Dog Game (Autodesk Fusion 360 design; units mm, degrees)
description: Spur Gear; Module: 1.5; Num Teeth: 32; Pressure Angle: 20.0; Backlash: 0.15 mm
description: Spur Gear; Module: 1.5; Num Teeth: 16; Pressure Angle: 20.0; Backlash: 0.15 mm
Autodesk Fusion 360 part; units mm, degrees
sketch "Sketch1" plane through (0, 0, 0) normal (0, 0, 1) x (1, 0, 0) in component "Pipe"
  arc A0 (120, 0) -> (-43.6285, 111.788) centre (0, 0) ccw
  dimension "d9" = 120
  constraint coincident A0.centre origin
  measures "d9" radius of A0
pipe "Pipe1" add diameter 91 wall 3 path "Sketch1" along A0 makes body 1 in component "Pipe"
sketch "Sketch1 (2)" plane through (0, 0, 0) normal (0, 1, 0) x (1, 0, 0) in component "Wheel"
  circle A0 centre (0, -56.6188) radius 34
  line L0 (-12.5, -25) -> (12.5, -25)
  line L1 (-12.5, -15) -> (12.5, -15)
  line L2 (12.5, -15) -> (12.5, -5)
  line L3 (12.5, -5) -> (-12.5, -5)
  line L4 (-12.5, -5) -> (-12.5, -15)
  line L5 (-12.5, -15) -> (12.5, -5) construction
  line L6 (12.5, -15) -> (-12.5, -5) construction
  line L7 (-9.5, -15) -> (-8.0858, -13.5858)
  line L8 (-9.5, -15) -> (-6.1258, -15) construction
  line L9 (9.5, -15) -> (8.0858, -13.5858)
  line L10 (9.5, -15) -> (10.773, -15) construction
  line L11 (-8.0858, -13.5858) -> (8.0858, -13.5858)
  line L12 (-1.4142, -13.5858) -> (0, -12.1716)
  line L13 (-1.4142, -13.5858) -> (0.8453, -13.5858) construction
  line L14 (0, 0) -> (0, -140)
  line L15 (1.4142, -13.5858) -> (0, -12.1716)
  line L16 (1.4142, -13.5858) -> (3.4142, -13.5858) construction
  arc A1 (12.5, -25) -> (12.5, -15) centre (8.3467, -20) ccw
  line L17 (12.5, -5) -> (-12.5, -5)
  line L18 (-12.5, -5) -> (-12.5, 0)
  line L19 (-12.5, 0) -> (12.5, 0)
  line L20 (12.5, 0) -> (12.5, -5)
  arc A2 (-12.5, -15) -> (-12.5, -25) centre (-8.3467, -20) ccw
  point P0 (0, -10)
  dimension "d40" = 68
  dimension "d42" = 25
  dimension "d43" = 25
  dimension "d45" = 45
  dimension "d46" = 2
  dimension "d47" = 3
  dimension "d48" = 135
  dimension "d49" = 2
  dimension "d50" = 3
  dimension "d51" = 2
  dimension "d52" = 45
  dimension "d53" = 140
  dimension "d54" = 135
  dimension "d55" = 2
  dimension "d60" = 10
  dimension "d61" = 5
  dimension "d62" = 6.5
  dimension "d64" = 10
  dimension "d65" = 6.5
  constraint horizontal L0
  constraint coincident A0 L0.start
  constraint coincident A0 L0.end
  constraint horizontal L1
  constraint perpendicular L1 L2
  constraint parallel L1 L3
  constraint parallel L2 L4
  constraint coincident L5 P0
  constraint coincident L6 P0
  constraint vertical L14.start P0
  constraint horizontal L8
  constraint coincident L1 L7.start
  constraint horizontal L10
  constraint coincident L1 L9.start
  constraint horizontal L13
  constraint coincident L11 L12.start
  constraint vertical L14
  constraint coincident L14.start origin
  constraint coincident L12.end L14
  constraint horizontal L16
  constraint coincident L11 L15.start
  constraint coincident L14 L12.end
  constraint coincident A0.centre L14
  constraint horizontal L17
  constraint vertical L18
  constraint horizontal L19
  constraint vertical L20
  constraint coincident L14.start L19
  measures "d40" diameter of A0
  measures "d42" distance of L0.start L0.end
  measures "d43" distance of L2.end L3.end
  measures "d45" angle of L7 L8
  measures "d46" distance of L7.start L7.end
  measures "d47" distance of L1.start L7.start
  measures "d48" angle of L9 L10
  measures "d49" distance of L9.start L9.end
  measures "d50" distance of L1.end L9.start
  measures "d51" distance of L12.start L12.end
  measures "d52" angle of L12 L13
  measures "d53" distance of L14.start L14.end
  measures "d54" angle of L15 L16
  measures "d55" distance of L15.start L12.end
  measures "d60" distance of L0 L1
  measures "d61" distance of L2.end L19.end
  measures "d62" radius of A1
  measures "d64" distance of L1.start L3.end
  measures "d65" radius of A2
revolve "Revolve1" add sketch "Sketch1 (2)" angle 360 about axis through (1.75, 0, 0) along (1, 0, 0) separate body contours L1 L2 L3 L9 L11 L14 L15 L17 | L3 L14 L17 L19 L20 | L1 L3 L4 L7 L11 L12 L14 L17 | L3 L14 L17 L18 L19 makes body 2 in component "Wheel"
revolve "Revolve2" add sketch "Sketch1 (2)" angle 360 about axis through (1.75, 0, 0) along (1, 0, 0) separate body contours A0 L1 L14 A1 | A0 L1 L14 A2 | L1 L9 L11 L14 | L1 L7 L11 L14 | L11 L14 L15 | L11 L12 L14 makes body 3 in component "Wheel"
fillet "Fillet1" radius 4.5 2 edges at (12.5, -9.0404, -23.3082) (-12.5, -9.0404, -23.3082) on bodies 3 in component "Wheel"
sketch "Sketch2" plane through (12.5, 0, 0) normal (1, 0, 0) x (0, 1, 0) in component "Wheel"
  circle A0 centre (0, 0) radius 15
  circle A1 centre (0, 0) radius 4
  circle A2 centre (0, 0) radius 7.5
  dimension "d68" = 8
  dimension "d69" = 15
  constraint concentric A0 A1
  constraint concentric A0 A2
  measures "d68" diameter of A1
  measures "d69" diameter of A2
extrude "Extrude1" cut sketch "Sketch2" against normal blind 40 contours A1 bodies 2 in component "Wheel"
extrude "Extrude2" add sketch "Sketch2" along normal blind 10 contours A2 bodies 2 in component "Wheel"
sketch "Sketch3" plane through (0, 0, 0) normal (0, 1, 0) x (1, 0, 0) in component "Wheel"
  line L0 (20, -2.5) -> (15, -2.5)
  line L1 (15, -2.5) -> (15, 2.5)
  line L2 (15, 2.5) -> (20, 2.5)
  line L3 (20, 2.5) -> (20, -2.5)
  line L4 (22.5, -7.5) -> (22.5, 7.5)
  circle A0 centre (17.5, 0) radius 1.5
  line L5 (0, 0) -> (31.5, 0)
  dimension "d74" = 5
  dimension "d75" = 5
  dimension "d76" = 2.5
  dimension "d77" = 3
  dimension "d85" = 2.5
  dimension "d86" = 2.5
  constraint horizontal L0
  constraint vertical L1
  constraint horizontal L2
  constraint vertical L3
  constraint coincident L5.start origin
  constraint perpendicular L3 L5
  constraint coincident A0.centre L5
  measures "d74" distance of L0.start L0.end
  measures "d75" distance of L0.start L2.end
  measures "d76" distance of L3 L4
  measures "d77" diameter of A0
  measures "d85" distance of L0 L5
  measures "d86" distance of L1 A0.centre
extrude "Extrude3" cut sketch "Sketch3" along normal blind 2 from surface at 6.7 bodies 2 in component "Wheel"
extrude "Extrude4" cut sketch "Sketch3" along normal blind 2 from surface at -8.7 bodies 2 in component "Wheel"
extrude "Extrude5" cut sketch "Sketch3" along normal mid plane 40 contours A0 L5 | A0 L5 bodies 2 in component "Wheel"
fillet "Fillet2" radius 2.5 1 edges at (12.5, -6.9925, 2.7121) on bodies 2 in component "Wheel"
sketch "Sketch1 (3)" plane through (0, 0, 0) normal (0, 0, 1) x (1, 0, 0) in component "Motor Connection"
  circle A0 centre (0, 0) radius 3.75
  circle A1 centre (0, 0) radius 6
  line L0 (-20.0347, 2.5) -> (19.9653, 2.5)
  line L1 (-1, 0) -> (1, 0)
  line L2 (1, 0) -> (1, -13.1685)
  line L3 (1, -13.1685) -> (-1, -13.1685)
  line L4 (-1, -13.1685) -> (-1, 0)
  circle A2 centre (0, 0) radius 4
  dimension "d1_1" = 7.5
  dimension "d2_1" = 12
  dimension "d3_1" = 40
  dimension "d4_1" = 2.5
  dimension "d5_1" = 2
  dimension "d95" = 8
  constraint coincident A0.centre A1.centre
  constraint horizontal L0
  constraint horizontal L1
  constraint vertical L2
  constraint horizontal L3
  constraint vertical L4
  constraint midpoint A0.centre L1
  measures "d1_1" diameter of A0
  measures "d2_1" diameter of A1
  measures "d3_1" distance of L0.start L0.end
  measures "d4_1" distance of A0.centre L0
  measures "d5_1" distance of L2.end L3.end
  measures "d95" diameter of A2
extrude "Extrude1'" add sketch "Sketch1 (3)" along normal blind 12.5 separate body contours A0 L0 L2 A2 | A0 L0 | A0 L0 A2 | A0 L0 L4 A2 | A1 L0 A2 | A1 L0 L2 A2 | A1 L0 L4 A2 makes body 4 in component "Motor Connection"
extrude "Extrude9" add sketch "Sketch1 (3)" along normal blind 12 from surface at 12 contours A1 L0 A2 | A1 L0 L2 A2 | A1 L0 L4 A2 bodies 4 in component "Motor Connection"
sketch "Sketch4" plane through (0, 0, 0) normal (1, 0, 0) x (0, 1, 0) in component "Motor Connection"
  line L0 (2.5, 20.5) -> (-2.5, 20.5)
  line L1 (-2.5, 20.5) -> (-2.5, 15.5)
  line L2 (-2.5, 15.5) -> (2.5, 15.5)
  line L3 (2.5, 15.5) -> (2.5, 20.5)
  line L4 (2.5, 20.5) -> (-2.5, 15.5) construction
  line L5 (-2.5, 20.5) -> (2.5, 15.5) construction
  line L6 (6, 24) -> (-5.9161, 24)
  circle A0 centre (0, 18) radius 1.5
  point P0 (0, 18)
  dimension "d99" = 5
  dimension "d100" = 5
  dimension "d101" = 3.5
  dimension "d102" = 3
  constraint horizontal L0
  constraint perpendicular L0 L1
  constraint parallel L0 L2
  constraint parallel L1 L3
  constraint coincident L4 P0
  constraint coincident L5 P0
  constraint coincident P0 A0.centre
  measures "d99" distance of L1.end L2.end
  measures "d100" distance of L0.end L1.end
  measures "d101" distance of L0 L6
  measures "d102" diameter of A0
extrude "Extrude10" cut sketch "Sketch4" along normal blind 2 from surface at 5.3 contours L0 L1 L2 L3 | A0 bodies 4 in component "Motor Connection"
extrude "Extrude11" cut sketch "Sketch4" along normal blind 2 from surface at -7.3 contours L0 L1 L2 L3 | A0 bodies 4 in component "Motor Connection"
extrude "Extrude12" cut sketch "Sketch4" along normal mid plane 40 contours A0 bodies 4 in component "Motor Connection"
sketch "Sketch1 (4)" plane through (0, 0, 0) normal (1, 0, 0) x (0, 1, 0) in component "Motor"
  circle A0 centre (0, 0) radius 17.9
  circle A1 centre (0, 0) radius 6.6
  circle A2 centre (12.5, 0) radius 1.5
  circle A3 centre (-12.5, 0) radius 1.5
  dimension "d111" = 35.8
  dimension "d112" = 13.2
  dimension "d113" = 3
  dimension "d114" = 12.5
  dimension "d115" = 3
  dimension "d116" = 12.5
  constraint coincident A0.centre A1.centre
  measures "d111" diameter of A0
  measures "d112" diameter of A1
  measures "d113" diameter of A2
  measures "d114" distance of A0.centre A2.centre
  measures "d115" diameter of A3
  measures "d116" distance of A0.centre A3.centre
extrude "Extrude1''" add sketch "Sketch1 (4)" along normal blind 58 separate body contours A0 | A1 | A2 | A3 makes body 5 in component "Motor"
extrude "Extrude2'" cut sketch "Sketch1 (4)" along normal blind 3 contours A2 | A3 bodies 5 in component "Motor"
extrude "Extrude3'" add sketch "Sketch1 (4)" against normal blind 4 contours A1 bodies 5 in component "Motor"
sketch "Sketch1 (5)" plane through (0, 0, 0) normal (1, 0, 0) x (0, 1, 0) in component "Motor Stand"
  line L0 (30, 30) -> (-100, 30)
  line L1 (-100, 30) -> (-100, -30)
  line L2 (-100, -30) -> (30, -30)
  line L3 (30, -30) -> (30, 30)
  circle A0 centre (0, 0) radius 6.6
  circle A1 centre (-12.5, 0) radius 1.5
  circle A2 centre (12.5, 0) radius 1.5
  point P0 (12.5, 0)
  dimension "d123" = 130
  dimension "d124" = 60
  dimension "d125" = 30
  dimension "d126" = 30
  constraint horizontal L0
  constraint vertical L1
  constraint horizontal L2
  constraint vertical L3
  measures "d123" distance of L0.start L0.end
  measures "d124" distance of L0.start L2.end
  measures "d125" distance of A0.centre L2
  measures "d126" distance of A0.centre L3
extrude "Extrude1'''" add sketch "Sketch1 (5)" against normal blind 4 separate body makes body 6 in component "Motor Stand"
sketch "Sketch1 (6)" plane through (0, 0, 0) normal (0, 0, 1) x (1, 0, 0) in component "Spur Gear (32 teeth) (1)"
  circle A0 centre (0, 0) radius 22.1492
  circle A1 centre (0, 0) radius 4
extrude "Extrude1''''" add sketch "Sketch1 (6)" along normal blind 5 separate body makes body 7 in component "Spur Gear (32 teeth) (1)"
sketch "Sketch2 (2)" plane through (0, 0, 0) normal (0, 0, 1) x (1, 0, 0) in component "Spur Gear (32 teeth) (1)"
  spline S0 degree 5 poles (22.5087, -1.407) (22.5173, -1.4076) (22.5344, -1.4084) (22.5602, -1.4091) (22.5946, -1.4089) (22.6376, -1.4072) (22.6806, -1.4043) (22.7236, -1.4007) (22.7667, -1.3967) (22.8098, -1.3925) (22.8528, -1.388) (22.8959, -1.3832) (22.939, -1.3779) (22.9821, -1.372) (23.0251, -1.3657) (23.0682, -1.3588) (23.1113, -1.3515) (23.1543, -1.3439) (23.1974, -1.3359) (23.2405, -1.3276) (23.2835, -1.319) (23.3265, -1.3102) (23.3695, -1.301) (23.4126, -1.2914) (23.4556, -1.2816) (23.4985, -1.2714) (23.5415, -1.2609) (23.5845, -1.2501) (23.6274, -1.2391) (23.6703, -1.2277) (23.7133, -1.2162) (23.7562, -1.2043) (23.799, -1.1922) (23.8419, -1.1798) (23.8847, -1.1671) (23.9276, -1.1542) (23.9704, -1.141) (24.0132, -1.1276) (24.0559, -1.1139) (24.0987, -1.1) (24.1414, -1.0859) (24.1841, -1.0715) (24.2268, -1.0568) (24.2695, -1.042) (24.3121, -1.0269) (24.3547, -1.0115) (24.3973, -0.996) (24.4399, -0.9802) (24.4824, -0.9642) (24.5249, -0.948) (24.5674, -0.9315) (24.6099, -0.9149) (24.6523, -0.898) (24.6947, -0.8809) (24.7371, -0.8636) (24.7794, -0.8461) (24.8218, -0.8284) (24.8641, -0.8104) (24.9063, -0.7923) (24.9486, -0.774) (24.9908, -0.7554) (25.0329, -0.7367) (25.0751, -0.7177) (25.1172, -0.6986) (25.1593, -0.6792) (25.2013, -0.6597) (25.2434, -0.6399) (25.2853, -0.62) (25.3273, -0.5999) (25.3692, -0.5796) (25.4111, -0.5591) (25.4446, -0.5425) (25.4697, -0.53) (25.4864, -0.5216) (25.4947, -0.5174) knots 0 0 0 0 0 0 0.01428571 0.02857143 0.04285714 0.05714286 0.07142857 0.08571429 0.1 0.11428571 0.12857143 0.14285714 0.15714286 0.17142857 0.18571429 0.2 0.21428571 0.22857143 0.24285714 0.25714286 0.27142857 0.28571429 0.3 0.31428571 0.32857143 0.34285714 0.35714286 0.37142857 0.38571429 0.4 0.41428571 0.42857143 0.44285714 0.45714286 0.47142857 0.48571429 0.5 0.51428571 0.52857143 0.54285714 0.55714286 0.57142857 0.58571429 0.6 0.61428571 0.62857143 0.64285714 0.65714286 0.67142857 0.68571429 0.7 0.71428571 0.72857143 0.74285714 0.75714286 0.77142857 0.78571429 0.8 0.81428571 0.82857143 0.84285714 0.85714286 0.87142857 0.88571429 0.9 0.91428571 0.92857143 0.94285714 0.95714286 0.97142857 0.98571429 1 1 1 1 1 1
  spline S1 degree 5 poles (22.5087, 1.407) (22.5173, 1.4076) (22.5344, 1.4084) (22.5602, 1.4091) (22.5946, 1.4089) (22.6376, 1.4072) (22.6806, 1.4043) (22.7236, 1.4007) (22.7667, 1.3967) (22.8098, 1.3925) (22.8528, 1.388) (22.8959, 1.3832) (22.939, 1.3779) (22.9821, 1.372) (23.0251, 1.3657) (23.0682, 1.3588) (23.1113, 1.3515) (23.1543, 1.3439) (23.1974, 1.3359) (23.2405, 1.3276) (23.2835, 1.319) (23.3265, 1.3102) (23.3695, 1.301) (23.4126, 1.2914) (23.4556, 1.2816) (23.4985, 1.2714) (23.5415, 1.2609) (23.5845, 1.2501) (23.6274, 1.2391) (23.6703, 1.2277) (23.7133, 1.2162) (23.7562, 1.2043) (23.799, 1.1922) (23.8419, 1.1798) (23.8847, 1.1671) (23.9276, 1.1542) (23.9704, 1.141) (24.0132, 1.1276) (24.0559, 1.1139) (24.0987, 1.1) (24.1414, 1.0859) (24.1841, 1.0715) (24.2268, 1.0568) (24.2695, 1.042) (24.3121, 1.0269) (24.3547, 1.0115) (24.3973, 0.996) (24.4399, 0.9802) (24.4824, 0.9642) (24.5249, 0.948) (24.5674, 0.9315) (24.6099, 0.9149) (24.6523, 0.898) (24.6947, 0.8809) (24.7371, 0.8636) (24.7794, 0.8461) (24.8218, 0.8284) (24.8641, 0.8104) (24.9063, 0.7923) (24.9486, 0.774) (24.9908, 0.7554) (25.0329, 0.7367) (25.0751, 0.7177) (25.1172, 0.6986) (25.1593, 0.6792) (25.2013, 0.6597) (25.2434, 0.6399) (25.2853, 0.62) (25.3273, 0.5999) (25.3692, 0.5796) (25.4111, 0.5591) (25.4446, 0.5425) (25.4697, 0.53) (25.4864, 0.5216) (25.4947, 0.5174) knots 0 0 0 0 0 0 0.01428571 0.02857143 0.04285714 0.05714286 0.07142857 0.08571429 0.1 0.11428571 0.12857143 0.14285714 0.15714286 0.17142857 0.18571429 0.2 0.21428571 0.22857143 0.24285714 0.25714286 0.27142857 0.28571429 0.3 0.31428571 0.32857143 0.34285714 0.35714286 0.37142857 0.38571429 0.4 0.41428571 0.42857143 0.44285714 0.45714286 0.47142857 0.48571429 0.5 0.51428571 0.52857143 0.54285714 0.55714286 0.57142857 0.58571429 0.6 0.61428571 0.62857143 0.64285714 0.65714286 0.67142857 0.68571429 0.7 0.71428571 0.72857143 0.74285714 0.75714286 0.77142857 0.78571429 0.8 0.81428571 0.82857143 0.84285714 0.85714286 0.87142857 0.88571429 0.9 0.91428571 0.92857143 0.94285714 0.95714286 0.97142857 0.98571429 1 1 1 1 1 1
  arc A0 (25.4947, -0.5174) -> (25.4947, 0.5174) centre (0, 0) ccw
  line L0 (22.0961, -1.3819) -> (22.5087, -1.407)
  line L1 (22.0961, 1.3819) -> (22.5087, 1.407)
  line L2 (22.0961, -1.3819) -> (22.0961, 1.3819)
  point P0 (22.72, -1.4009)
  point P1 (22.9323, -1.3786)
  point P2 (23.1451, -1.3454)
  point P3 (23.3584, -1.3033)
  point P4 (23.572, -1.2532)
  point P5 (23.7857, -1.1959)
  point P6 (23.9996, -1.1318)
  point P7 (24.2136, -1.0613)
  point P8 (24.4275, -0.9848)
  point P9 (24.6414, -0.9023)
  point P10 (24.8551, -0.8142)
  point P11 (25.0686, -0.7206)
  point P12 (25.2818, -0.6216)
  point P13 (22.72, 1.4009)
  point P14 (22.9323, 1.3786)
  point P15 (23.1451, 1.3454)
  point P16 (23.3584, 1.3033)
  point P17 (23.572, 1.2532)
  point P18 (23.7857, 1.1959)
  point P19 (23.9996, 1.1318)
  point P20 (24.2136, 1.0613)
  point P21 (24.4275, 0.9848)
  point P22 (24.6414, 0.9023)
  point P23 (24.8551, 0.8142)
  point P24 (25.0686, 0.7206)
  point P25 (25.2818, 0.6216)
extrude "Extrude2''" add sketch "Sketch2 (2)" along normal blind 5 bodies 7 in component "Spur Gear (32 teeth) (1)"
fillet "Fillet1'" radius 0.35 2 edges at (22.106, -1.3825, 2.5) (22.106, 1.3825, 2.5) on bodies 7 in component "Spur Gear (32 teeth) (1)"
pattern_circular "C-Pattern1" count 32 over 360 about axis through (0, 0, 0) along (0, 0, 1) of "Extrude2''", "Fillet1'" in component "Spur Gear (32 teeth) (1)"
sketch "Sketch3 (2)" plane through (0, 0, 0) normal (0, 0, 1) x (1, 0, 0) in component "Spur Gear (32 teeth) (1)"
  circle A0 centre (0, 0) radius 24 construction
sketch "Sketch1 (7)" plane through (0, 0, 0) normal (0, 0, 1) x (1, 0, 0) in component "Spur Gear (16 teeth) (1)"
  circle A0 centre (0, 0) radius 10.1492
  circle A1 centre (0, 0) radius 4
extrude "Extrude1'''''" add sketch "Sketch1 (7)" along normal blind 5 separate body makes body 8 in component "Spur Gear (16 teeth) (1)"
sketch "Sketch2 (3)" plane through (0, 0, 0) normal (0, 0, 1) x (1, 0, 0) in component "Spur Gear (16 teeth) (1)"
  spline S0 degree 5 poles (11.2082, -1.2374) (11.2147, -1.2381) (11.2277, -1.2393) (11.2473, -1.2406) (11.2734, -1.2413) (11.3061, -1.2407) (11.3389, -1.2391) (11.3717, -1.2368) (11.4045, -1.2342) (11.4374, -1.2313) (11.4703, -1.2282) (11.5033, -1.2247) (11.5362, -1.2208) (11.5691, -1.2164) (11.6021, -1.2114) (11.6351, -1.206) (11.6681, -1.2002) (11.7011, -1.194) (11.7341, -1.1876) (11.7671, -1.1808) (11.8001, -1.1738) (11.8331, -1.1665) (11.8661, -1.1588) (11.8991, -1.1508) (11.9321, -1.1425) (11.9651, -1.1339) (11.9981, -1.125) (12.031, -1.1159) (12.064, -1.1064) (12.097, -1.0967) (12.1299, -1.0867) (12.1629, -1.0765) (12.1958, -1.066) (12.2287, -1.0552) (12.2616, -1.0442) (12.2945, -1.0329) (12.3273, -1.0214) (12.3602, -1.0096) (12.393, -0.9975) (12.4258, -0.9853) (12.4586, -0.9728) (12.4913, -0.96) (12.5241, -0.9471) (12.5568, -0.9338) (12.5895, -0.9204) (12.6221, -0.9067) (12.6548, -0.8928) (12.6874, -0.8787) (12.72, -0.8644) (12.7526, -0.8498) (12.7851, -0.835) (12.8176, -0.82) (12.8501, -0.8048) (12.8825, -0.7894) (12.9149, -0.7737) (12.9473, -0.7579) (12.9797, -0.7418) (13.012, -0.7255) (13.0443, -0.709) (13.0765, -0.6923) (13.1087, -0.6754) (13.1409, -0.6583) (13.1731, -0.641) (13.2052, -0.6235) (13.2372, -0.6058) (13.2692, -0.5879) (13.3012, -0.5698) (13.3332, -0.5515) (13.3651, -0.533) (13.3969, -0.5143) (13.4288, -0.4954) (13.4542, -0.4801) (13.4732, -0.4686) (13.4859, -0.4609) (13.4923, -0.457) knots 0 0 0 0 0 0 0.01428571 0.02857143 0.04285714 0.05714286 0.07142857 0.08571429 0.1 0.11428571 0.12857143 0.14285714 0.15714286 0.17142857 0.18571429 0.2 0.21428571 0.22857143 0.24285714 0.25714286 0.27142857 0.28571429 0.3 0.31428571 0.32857143 0.34285714 0.35714286 0.37142857 0.38571429 0.4 0.41428571 0.42857143 0.44285714 0.45714286 0.47142857 0.48571429 0.5 0.51428571 0.52857143 0.54285714 0.55714286 0.57142857 0.58571429 0.6 0.61428571 0.62857143 0.64285714 0.65714286 0.67142857 0.68571429 0.7 0.71428571 0.72857143 0.74285714 0.75714286 0.77142857 0.78571429 0.8 0.81428571 0.82857143 0.84285714 0.85714286 0.87142857 0.88571429 0.9 0.91428571 0.92857143 0.94285714 0.95714286 0.97142857 0.98571429 1 1 1 1 1 1
  spline S1 degree 5 poles (11.2082, 1.2374) (11.2147, 1.2381) (11.2277, 1.2393) (11.2473, 1.2406) (11.2734, 1.2413) (11.3061, 1.2407) (11.3389, 1.2391) (11.3717, 1.2368) (11.4045, 1.2342) (11.4374, 1.2313) (11.4703, 1.2282) (11.5033, 1.2247) (11.5362, 1.2208) (11.5691, 1.2164) (11.6021, 1.2114) (11.6351, 1.206) (11.6681, 1.2002) (11.7011, 1.194) (11.7341, 1.1876) (11.7671, 1.1808) (11.8001, 1.1738) (11.8331, 1.1665) (11.8661, 1.1588) (11.8991, 1.1508) (11.9321, 1.1425) (11.9651, 1.1339) (11.9981, 1.125) (12.031, 1.1159) (12.064, 1.1064) (12.097, 1.0967) (12.1299, 1.0867) (12.1629, 1.0765) (12.1958, 1.066) (12.2287, 1.0552) (12.2616, 1.0442) (12.2945, 1.0329) (12.3273, 1.0214) (12.3602, 1.0096) (12.393, 0.9975) (12.4258, 0.9853) (12.4586, 0.9728) (12.4913, 0.96) (12.5241, 0.9471) (12.5568, 0.9338) (12.5895, 0.9204) (12.6221, 0.9067) (12.6548, 0.8928) (12.6874, 0.8787) (12.72, 0.8644) (12.7526, 0.8498) (12.7851, 0.835) (12.8176, 0.82) (12.8501, 0.8048) (12.8825, 0.7894) (12.9149, 0.7737) (12.9473, 0.7579) (12.9797, 0.7418) (13.012, 0.7255) (13.0443, 0.709) (13.0765, 0.6923) (13.1087, 0.6754) (13.1409, 0.6583) (13.1731, 0.641) (13.2052, 0.6235) (13.2372, 0.6058) (13.2692, 0.5879) (13.3012, 0.5698) (13.3332, 0.5515) (13.3651, 0.533) (13.3969, 0.5143) (13.4288, 0.4954) (13.4542, 0.4801) (13.4732, 0.4686) (13.4859, 0.4609) (13.4923, 0.457) knots 0 0 0 0 0 0 0.01428571 0.02857143 0.04285714 0.05714286 0.07142857 0.08571429 0.1 0.11428571 0.12857143 0.14285714 0.15714286 0.17142857 0.18571429 0.2 0.21428571 0.22857143 0.24285714 0.25714286 0.27142857 0.28571429 0.3 0.31428571 0.32857143 0.34285714 0.35714286 0.37142857 0.38571429 0.4 0.41428571 0.42857143 0.44285714 0.45714286 0.47142857 0.48571429 0.5 0.51428571 0.52857143 0.54285714 0.55714286 0.57142857 0.58571429 0.6 0.61428571 0.62857143 0.64285714 0.65714286 0.67142857 0.68571429 0.7 0.71428571 0.72857143 0.74285714 0.75714286 0.77142857 0.78571429 0.8 0.81428571 0.82857143 0.84285714 0.85714286 0.87142857 0.88571429 0.9 0.91428571 0.92857143 0.94285714 0.95714286 0.97142857 0.98571429 1 1 1 1 1 1
  arc A0 (13.4923, -0.457) -> (13.4923, 0.457) centre (0, 0) ccw
  line L0 (10.078, -1.1137) -> (11.2082, -1.2374)
  line L1 (10.078, 1.1137) -> (11.2082, 1.2374)
  line L2 (10.078, -1.1137) -> (10.078, 1.1137)
  point P0 (11.368, -1.237)
  point P1 (11.5295, -1.2215)
  point P2 (11.6918, -1.1957)
  point P3 (11.8549, -1.1614)
  point P4 (12.0185, -1.1193)
  point P5 (12.1824, -1.0702)
  point P6 (12.3466, -1.0144)
  point P7 (12.5108, -0.9523)
  point P8 (12.675, -0.884)
  point P9 (12.8391, -0.8099)
  point P10 (13.003, -0.73)
  point P11 (13.1666, -0.6445)
  point P12 (13.3297, -0.5534)
  point P13 (11.368, 1.237)
  point P14 (11.5295, 1.2215)
  point P15 (11.6918, 1.1957)
  point P16 (11.8549, 1.1614)
  point P17 (12.0185, 1.1193)
  point P18 (12.1824, 1.0702)
  point P19 (12.3466, 1.0144)
  point P20 (12.5108, 0.9523)
  point P21 (12.675, 0.884)
  point P22 (12.8391, 0.8099)
  point P23 (13.003, 0.73)
  point P24 (13.1666, 0.6445)
  point P25 (13.3297, 0.5534)
extrude "Extrude2'''" add sketch "Sketch2 (3)" along normal blind 5 bodies 8 in component "Spur Gear (16 teeth) (1)"
fillet "Fillet1''" radius 0.175 2 edges at (10.0878, -1.1148, 2.5) (10.0878, 1.1148, 2.5) on bodies 8 in component "Spur Gear (16 teeth) (1)"
pattern_circular "C-Pattern1'" count 16 over 360 about axis through (0, 0, 0) along (0, 0, 1) of "Extrude2'''", "Fillet1''" in component "Spur Gear (16 teeth) (1)"
sketch "Sketch3 (3)" plane through (0, 0, 0) normal (0, 0, 1) x (1, 0, 0) in component "Spur Gear (16 teeth) (1)"
  circle A0 centre (0, 0) radius 12 construction
sketch "Sketch1 (8)" plane through (0, 0, 0) normal (0, 0, 1) x (1, 0, 0) in component "Spur Gear (32 teeth)"
  circle A0 centre (0, 0) radius 22.1492
  circle A1 centre (0, 0) radius 4
extrude "Extrude1''''''" add sketch "Sketch1 (8)" along normal blind 5 separate body makes body 9 in component "Spur Gear (32 teeth)"
sketch "Sketch2 (4)" plane through (0, 0, 0) normal (0, 0, 1) x (1, 0, 0) in component "Spur Gear (32 teeth)"
  spline S0 degree 5 poles (22.5087, -1.407) (22.5173, -1.4076) (22.5344, -1.4084) (22.5602, -1.4091) (22.5946, -1.4089) (22.6376, -1.4072) (22.6806, -1.4043) (22.7236, -1.4007) (22.7667, -1.3967) (22.8098, -1.3925) (22.8528, -1.388) (22.8959, -1.3832) (22.939, -1.3779) (22.9821, -1.372) (23.0251, -1.3657) (23.0682, -1.3588) (23.1113, -1.3515) (23.1543, -1.3439) (23.1974, -1.3359) (23.2405, -1.3276) (23.2835, -1.319) (23.3265, -1.3102) (23.3695, -1.301) (23.4126, -1.2914) (23.4556, -1.2816) (23.4985, -1.2714) (23.5415, -1.2609) (23.5845, -1.2501) (23.6274, -1.2391) (23.6703, -1.2277) (23.7133, -1.2162) (23.7562, -1.2043) (23.799, -1.1922) (23.8419, -1.1798) (23.8847, -1.1671) (23.9276, -1.1542) (23.9704, -1.141) (24.0132, -1.1276) (24.0559, -1.1139) (24.0987, -1.1) (24.1414, -1.0859) (24.1841, -1.0715) (24.2268, -1.0568) (24.2695, -1.042) (24.3121, -1.0269) (24.3547, -1.0115) (24.3973, -0.996) (24.4399, -0.9802) (24.4824, -0.9642) (24.5249, -0.948) (24.5674, -0.9315) (24.6099, -0.9149) (24.6523, -0.898) (24.6947, -0.8809) (24.7371, -0.8636) (24.7794, -0.8461) (24.8218, -0.8284) (24.8641, -0.8104) (24.9063, -0.7923) (24.9486, -0.774) (24.9908, -0.7554) (25.0329, -0.7367) (25.0751, -0.7177) (25.1172, -0.6986) (25.1593, -0.6792) (25.2013, -0.6597) (25.2434, -0.6399) (25.2853, -0.62) (25.3273, -0.5999) (25.3692, -0.5796) (25.4111, -0.5591) (25.4446, -0.5425) (25.4697, -0.53) (25.4864, -0.5216) (25.4947, -0.5174) knots 0 0 0 0 0 0 0.01428571 0.02857143 0.04285714 0.05714286 0.07142857 0.08571429 0.1 0.11428571 0.12857143 0.14285714 0.15714286 0.17142857 0.18571429 0.2 0.21428571 0.22857143 0.24285714 0.25714286 0.27142857 0.28571429 0.3 0.31428571 0.32857143 0.34285714 0.35714286 0.37142857 0.38571429 0.4 0.41428571 0.42857143 0.44285714 0.45714286 0.47142857 0.48571429 0.5 0.51428571 0.52857143 0.54285714 0.55714286 0.57142857 0.58571429 0.6 0.61428571 0.62857143 0.64285714 0.65714286 0.67142857 0.68571429 0.7 0.71428571 0.72857143 0.74285714 0.75714286 0.77142857 0.78571429 0.8 0.81428571 0.82857143 0.84285714 0.85714286 0.87142857 0.88571429 0.9 0.91428571 0.92857143 0.94285714 0.95714286 0.97142857 0.98571429 1 1 1 1 1 1
  spline S1 degree 5 poles (22.5087, 1.407) (22.5173, 1.4076) (22.5344, 1.4084) (22.5602, 1.4091) (22.5946, 1.4089) (22.6376, 1.4072) (22.6806, 1.4043) (22.7236, 1.4007) (22.7667, 1.3967) (22.8098, 1.3925) (22.8528, 1.388) (22.8959, 1.3832) (22.939, 1.3779) (22.9821, 1.372) (23.0251, 1.3657) (23.0682, 1.3588) (23.1113, 1.3515) (23.1543, 1.3439) (23.1974, 1.3359) (23.2405, 1.3276) (23.2835, 1.319) (23.3265, 1.3102) (23.3695, 1.301) (23.4126, 1.2914) (23.4556, 1.2816) (23.4985, 1.2714) (23.5415, 1.2609) (23.5845, 1.2501) (23.6274, 1.2391) (23.6703, 1.2277) (23.7133, 1.2162) (23.7562, 1.2043) (23.799, 1.1922) (23.8419, 1.1798) (23.8847, 1.1671) (23.9276, 1.1542) (23.9704, 1.141) (24.0132, 1.1276) (24.0559, 1.1139) (24.0987, 1.1) (24.1414, 1.0859) (24.1841, 1.0715) (24.2268, 1.0568) (24.2695, 1.042) (24.3121, 1.0269) (24.3547, 1.0115) (24.3973, 0.996) (24.4399, 0.9802) (24.4824, 0.9642) (24.5249, 0.948) (24.5674, 0.9315) (24.6099, 0.9149) (24.6523, 0.898) (24.6947, 0.8809) (24.7371, 0.8636) (24.7794, 0.8461) (24.8218, 0.8284) (24.8641, 0.8104) (24.9063, 0.7923) (24.9486, 0.774) (24.9908, 0.7554) (25.0329, 0.7367) (25.0751, 0.7177) (25.1172, 0.6986) (25.1593, 0.6792) (25.2013, 0.6597) (25.2434, 0.6399) (25.2853, 0.62) (25.3273, 0.5999) (25.3692, 0.5796) (25.4111, 0.5591) (25.4446, 0.5425) (25.4697, 0.53) (25.4864, 0.5216) (25.4947, 0.5174) knots 0 0 0 0 0 0 0.01428571 0.02857143 0.04285714 0.05714286 0.07142857 0.08571429 0.1 0.11428571 0.12857143 0.14285714 0.15714286 0.17142857 0.18571429 0.2 0.21428571 0.22857143 0.24285714 0.25714286 0.27142857 0.28571429 0.3 0.31428571 0.32857143 0.34285714 0.35714286 0.37142857 0.38571429 0.4 0.41428571 0.42857143 0.44285714 0.45714286 0.47142857 0.48571429 0.5 0.51428571 0.52857143 0.54285714 0.55714286 0.57142857 0.58571429 0.6 0.61428571 0.62857143 0.64285714 0.65714286 0.67142857 0.68571429 0.7 0.71428571 0.72857143 0.74285714 0.75714286 0.77142857 0.78571429 0.8 0.81428571 0.82857143 0.84285714 0.85714286 0.87142857 0.88571429 0.9 0.91428571 0.92857143 0.94285714 0.95714286 0.97142857 0.98571429 1 1 1 1 1 1
  arc A0 (25.4947, -0.5174) -> (25.4947, 0.5174) centre (0, 0) ccw
  line L0 (22.0961, -1.3819) -> (22.5087, -1.407)
  line L1 (22.0961, 1.3819) -> (22.5087, 1.407)
  line L2 (22.0961, -1.3819) -> (22.0961, 1.3819)
  point P0 (22.72, -1.4009)
  point P1 (22.9323, -1.3786)
  point P2 (23.1451, -1.3454)
  point P3 (23.3584, -1.3033)
  point P4 (23.572, -1.2532)
  point P5 (23.7857, -1.1959)
  point P6 (23.9996, -1.1318)
  point P7 (24.2136, -1.0613)
  point P8 (24.4275, -0.9848)
  point P9 (24.6414, -0.9023)
  point P10 (24.8551, -0.8142)
  point P11 (25.0686, -0.7206)
  point P12 (25.2818, -0.6216)
  point P13 (22.72, 1.4009)
  point P14 (22.9323, 1.3786)
  point P15 (23.1451, 1.3454)
  point P16 (23.3584, 1.3033)
  point P17 (23.572, 1.2532)
  point P18 (23.7857, 1.1959)
  point P19 (23.9996, 1.1318)
  point P20 (24.2136, 1.0613)
  point P21 (24.4275, 0.9848)
  point P22 (24.6414, 0.9023)
  point P23 (24.8551, 0.8142)
  point P24 (25.0686, 0.7206)
  point P25 (25.2818, 0.6216)
extrude "Extrude2''''" add sketch "Sketch2 (4)" along normal blind 5 bodies 9 in component "Spur Gear (32 teeth)"
fillet "Fillet1'''" radius 0.175 2 edges at (22.106, -1.3825, 2.5) (22.106, 1.3825, 2.5) on bodies 9 in component "Spur Gear (32 teeth)"
pattern_circular "C-Pattern1''" count 32 over 360 about axis through (0, 0, 0) along (0, 0, 1) of "Extrude2''''", "Fillet1'''" in component "Spur Gear (32 teeth)"
sketch "Sketch3 (4)" plane through (0, 0, 0) normal (0, 0, 1) x (1, 0, 0) in component "Spur Gear (32 teeth)"
  circle A0 centre (0, 0) radius 24 construction
sketch "Sketch1 (9)" plane through (0, 0, 0) normal (0, 0, 1) x (1, 0, 0) in component "Spur Gear (32 teeth) (2)"
  circle A0 centre (0, 0) radius 22.1492
  circle A1 centre (0, 0) radius 4
extrude "Extrude1'''''''" add sketch "Sketch1 (9)" along normal blind 5 separate body makes body 10 in component "Spur Gear (32 teeth) (2)"
sketch "Sketch2 (5)" plane through (0, 0, 0) normal (0, 0, 1) x (1, 0, 0) in component "Spur Gear (32 teeth) (2)"
  spline S0 degree 5 poles (22.5087, -1.407) (22.5173, -1.4076) (22.5344, -1.4084) (22.5602, -1.4091) (22.5946, -1.4089) (22.6376, -1.4072) (22.6806, -1.4043) (22.7236, -1.4007) (22.7667, -1.3967) (22.8098, -1.3925) (22.8528, -1.388) (22.8959, -1.3832) (22.939, -1.3779) (22.9821, -1.372) (23.0251, -1.3657) (23.0682, -1.3588) (23.1113, -1.3515) (23.1543, -1.3439) (23.1974, -1.3359) (23.2405, -1.3276) (23.2835, -1.319) (23.3265, -1.3102) (23.3695, -1.301) (23.4126, -1.2914) (23.4556, -1.2816) (23.4985, -1.2714) (23.5415, -1.2609) (23.5845, -1.2501) (23.6274, -1.2391) (23.6703, -1.2277) (23.7133, -1.2162) (23.7562, -1.2043) (23.799, -1.1922) (23.8419, -1.1798) (23.8847, -1.1671) (23.9276, -1.1542) (23.9704, -1.141) (24.0132, -1.1276) (24.0559, -1.1139) (24.0987, -1.1) (24.1414, -1.0859) (24.1841, -1.0715) (24.2268, -1.0568) (24.2695, -1.042) (24.3121, -1.0269) (24.3547, -1.0115) (24.3973, -0.996) (24.4399, -0.9802) (24.4824, -0.9642) (24.5249, -0.948) (24.5674, -0.9315) (24.6099, -0.9149) (24.6523, -0.898) (24.6947, -0.8809) (24.7371, -0.8636) (24.7794, -0.8461) (24.8218, -0.8284) (24.8641, -0.8104) (24.9063, -0.7923) (24.9486, -0.774) (24.9908, -0.7554) (25.0329, -0.7367) (25.0751, -0.7177) (25.1172, -0.6986) (25.1593, -0.6792) (25.2013, -0.6597) (25.2434, -0.6399) (25.2853, -0.62) (25.3273, -0.5999) (25.3692, -0.5796) (25.4111, -0.5591) (25.4446, -0.5425) (25.4697, -0.53) (25.4864, -0.5216) (25.4947, -0.5174) knots 0 0 0 0 0 0 0.01428571 0.02857143 0.04285714 0.05714286 0.07142857 0.08571429 0.1 0.11428571 0.12857143 0.14285714 0.15714286 0.17142857 0.18571429 0.2 0.21428571 0.22857143 0.24285714 0.25714286 0.27142857 0.28571429 0.3 0.31428571 0.32857143 0.34285714 0.35714286 0.37142857 0.38571429 0.4 0.41428571 0.42857143 0.44285714 0.45714286 0.47142857 0.48571429 0.5 0.51428571 0.52857143 0.54285714 0.55714286 0.57142857 0.58571429 0.6 0.61428571 0.62857143 0.64285714 0.65714286 0.67142857 0.68571429 0.7 0.71428571 0.72857143 0.74285714 0.75714286 0.77142857 0.78571429 0.8 0.81428571 0.82857143 0.84285714 0.85714286 0.87142857 0.88571429 0.9 0.91428571 0.92857143 0.94285714 0.95714286 0.97142857 0.98571429 1 1 1 1 1 1
  spline S1 degree 5 poles (22.5087, 1.407) (22.5173, 1.4076) (22.5344, 1.4084) (22.5602, 1.4091) (22.5946, 1.4089) (22.6376, 1.4072) (22.6806, 1.4043) (22.7236, 1.4007) (22.7667, 1.3967) (22.8098, 1.3925) (22.8528, 1.388) (22.8959, 1.3832) (22.939, 1.3779) (22.9821, 1.372) (23.0251, 1.3657) (23.0682, 1.3588) (23.1113, 1.3515) (23.1543, 1.3439) (23.1974, 1.3359) (23.2405, 1.3276) (23.2835, 1.319) (23.3265, 1.3102) (23.3695, 1.301) (23.4126, 1.2914) (23.4556, 1.2816) (23.4985, 1.2714) (23.5415, 1.2609) (23.5845, 1.2501) (23.6274, 1.2391) (23.6703, 1.2277) (23.7133, 1.2162) (23.7562, 1.2043) (23.799, 1.1922) (23.8419, 1.1798) (23.8847, 1.1671) (23.9276, 1.1542) (23.9704, 1.141) (24.0132, 1.1276) (24.0559, 1.1139) (24.0987, 1.1) (24.1414, 1.0859) (24.1841, 1.0715) (24.2268, 1.0568) (24.2695, 1.042) (24.3121, 1.0269) (24.3547, 1.0115) (24.3973, 0.996) (24.4399, 0.9802) (24.4824, 0.9642) (24.5249, 0.948) (24.5674, 0.9315) (24.6099, 0.9149) (24.6523, 0.898) (24.6947, 0.8809) (24.7371, 0.8636) (24.7794, 0.8461) (24.8218, 0.8284) (24.8641, 0.8104) (24.9063, 0.7923) (24.9486, 0.774) (24.9908, 0.7554) (25.0329, 0.7367) (25.0751, 0.7177) (25.1172, 0.6986) (25.1593, 0.6792) (25.2013, 0.6597) (25.2434, 0.6399) (25.2853, 0.62) (25.3273, 0.5999) (25.3692, 0.5796) (25.4111, 0.5591) (25.4446, 0.5425) (25.4697, 0.53) (25.4864, 0.5216) (25.4947, 0.5174) knots 0 0 0 0 0 0 0.01428571 0.02857143 0.04285714 0.05714286 0.07142857 0.08571429 0.1 0.11428571 0.12857143 0.14285714 0.15714286 0.17142857 0.18571429 0.2 0.21428571 0.22857143 0.24285714 0.25714286 0.27142857 0.28571429 0.3 0.31428571 0.32857143 0.34285714 0.35714286 0.37142857 0.38571429 0.4 0.41428571 0.42857143 0.44285714 0.45714286 0.47142857 0.48571429 0.5 0.51428571 0.52857143 0.54285714 0.55714286 0.57142857 0.58571429 0.6 0.61428571 0.62857143 0.64285714 0.65714286 0.67142857 0.68571429 0.7 0.71428571 0.72857143 0.74285714 0.75714286 0.77142857 0.78571429 0.8 0.81428571 0.82857143 0.84285714 0.85714286 0.87142857 0.88571429 0.9 0.91428571 0.92857143 0.94285714 0.95714286 0.97142857 0.98571429 1 1 1 1 1 1
  arc A0 (25.4947, -0.5174) -> (25.4947, 0.5174) centre (0, 0) ccw
  line L0 (22.0961, -1.3819) -> (22.5087, -1.407)
  line L1 (22.0961, 1.3819) -> (22.5087, 1.407)
  line L2 (22.0961, -1.3819) -> (22.0961, 1.3819)
  point P0 (22.72, -1.4009)
  point P1 (22.9323, -1.3786)
  point P2 (23.1451, -1.3454)
  point P3 (23.3584, -1.3033)
  point P4 (23.572, -1.2532)
  point P5 (23.7857, -1.1959)
  point P6 (23.9996, -1.1318)
  point P7 (24.2136, -1.0613)
  point P8 (24.4275, -0.9848)
  point P9 (24.6414, -0.9023)
  point P10 (24.8551, -0.8142)
  point P11 (25.0686, -0.7206)
  point P12 (25.2818, -0.6216)
  point P13 (22.72, 1.4009)
  point P14 (22.9323, 1.3786)
  point P15 (23.1451, 1.3454)
  point P16 (23.3584, 1.3033)
  point P17 (23.572, 1.2532)
  point P18 (23.7857, 1.1959)
  point P19 (23.9996, 1.1318)
  point P20 (24.2136, 1.0613)
  point P21 (24.4275, 0.9848)
  point P22 (24.6414, 0.9023)
  point P23 (24.8551, 0.8142)
  point P24 (25.0686, 0.7206)
  point P25 (25.2818, 0.6216)
extrude "Extrude2'''''" add sketch "Sketch2 (5)" along normal blind 5 bodies 10 in component "Spur Gear (32 teeth) (2)"
fillet "Fillet1''''" radius 0.175 2 edges at (22.106, -1.3825, 2.5) (22.106, 1.3825, 2.5) on bodies 10 in component "Spur Gear (32 teeth) (2)"
pattern_circular "C-Pattern1'''" count 32 over 360 about axis through (0, 0, 0) along (0, 0, 1) of "Extrude2'''''", "Fillet1''''" in component "Spur Gear (32 teeth) (2)"
sketch "Sketch3 (5)" plane through (0, 0, 0) normal (0, 0, 1) x (1, 0, 0) in component "Spur Gear (32 teeth) (2)"
  circle A0 centre (0, 0) radius 24 construction
sketch "Sketch3 (6)" plane through (-4, 0, 0) normal (-1, 0, 0) x (0, -1, 0) in component "Motor Stand"
  circle A0 centre (12.5, 0) radius 1.5
  circle A1 centre (0, 0) radius 6.6
  circle A2 centre (-12.5, 0) radius 1.5
  line L0 (-30, 30) -> (-30, -30)
  line L1 (-30, -30) -> (100, -30)
  line L2 (100, -30) -> (100, 30)
  line L3 (100, 30) -> (-30, 30)
  circle A3 centre (48, 0) radius 4
extrude "Extrude6" cut sketch "Sketch3 (6)" against normal blind 25 contours A3 sketch seen with x (1, 0, 0) y (0, 1, 0) z (0, 0, 1) at (-25, 55, 0) bodies 2 in component "Wheel"
extrude "Extrude3''" cut sketch "Sketch3 (6)" against normal blind 25 contours A3 bodies 6 in component "Motor Stand"
component "Pipe" placed x (1, 0, 0) y (0, 1, 0) z (0, 0, 1) at (0, 0, 0)
component "Wheel" placed x (1, 0, 0) y (0, 1, 0) z (0, 0, 1) at (25, -55, 0)
component "Motor Connection" placed x (1, 0, 0) y (0, 1, 0) z (0, 0, 1) at (0, 0, 0)
component "Motor" placed x (1, 0, 0) y (0, 1, 0) z (0, 0, 1) at (0, 0, 0)
component "Motor Stand" placed x (1, 0, 0) y (0, 1, 0) z (0, 0, 1) at (0, 0, 0)
component "Spur Gear (32 teeth) (1)" placed x (0, 0.09932, -0.995056) y (0, 0.995056, 0.09932) z (1, 0, 0) at (-9.5, -36, 0)
component "Spur Gear (16 teeth) (1)" placed x (0, 0, -1) y (0, 1, 0) z (1, 0, 0) at (-9.5, 0, 0)
component "Spur Gear (32 teeth)" placed x (0, 0, -1) y (0, 1, 0) z (1, 0, 0) at (-12.5, 0, 0)
component "Spur Gear (32 teeth) (2)" placed x (0, 0.097583, -0.995227) y (0, 0.995227, 0.097583) z (1, 0, 0) at (-12.5, -48, 0)
equation "taperAngle1 = 0.0 deg"
equation "Radius = 0.175 mm"
equation "countU = 32"
equation "taperAngle1_1 = 0.0 deg"
equation "Radius_1 = 0.175 mm"
equation "countU_1 = 32"
